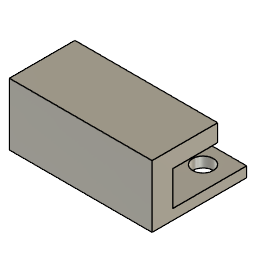
舵机固定 (Autodesk Fusion 360 design; units mm, degrees)
part number: 2025-10-23-15-03-21-135
part number: 2025-10-23-15-21-45-592
Autodesk Fusion 360 part; units mm, degrees
sketch "草图1" plane through (0, 0, 0) normal (0, 0, 1) x (1, 0, 0)
  circle A0 centre (0, 0) radius 1.5
  circle A1 centre (-14, 0) radius 1.5
  line L0 (-14, 0) -> (0, 0) construction
  line L1 (-7, 0) -> (-7, -17.5669) construction
  dimension "d1" = 3
  dimension "d2" = 14
  dimension "d3" = 3
  constraint coincident A0.centre L0.end
  constraint coincident A1.centre L0.start
  constraint horizontal L0
  constraint midpoint L0 L1.start
  constraint perpendicular L0 L1
  measures "d1" diameter of A0
  measures "d2" distance of A1.centre A0.centre
  measures "d3" diameter of A1
sketch "草图2" plane through (0, 0, 0) normal (0, 0, 1) x (1, 0, 0)
  line L0 (-17.3282, -10.7) -> (-17.3282, 3)
  line L1 (-17.3282, 3) -> (3.3282, 3)
  line L2 (3.3282, 3) -> (3.3282, -10.7)
  line L3 (-7, 0) -> (-7, -17.5669)
  line L4 (3.3282, -10.7) -> (-17.3282, -10.7)
  line L5 (-14, 0) -> (0, 0)
  dimension "d4" = 10.7
  dimension "d11" = 3
  constraint vertical L0
  constraint perpendicular L0 L1
  constraint perpendicular L1 L2
  constraint symmetric L0 L2 L3
  constraint perpendicular L0 L4
  measures "d4" distance of L4 L5
  measures "d11" distance of L5.end L1
extrude "拉伸1" add sketch "草图2" along normal blind 1.5 in component "Component'"
extrude "拉伸2" cut sketch "草图1" along normal blind 4 in component "Component'"
sketch "草图4" plane through (0, 0, 1.5) normal (0, 0, 1) x (-1, 0, 0)
  circle A0 centre (14, 0) radius 1.5
  circle A1 centre (0, 0) radius 1.5
  line L0 (-3.3282, 10.7) -> (-3.3282, -3)
  line L1 (-3.3282, -3) -> (17.3282, -3)
  line L2 (17.3282, -3) -> (17.3282, 10.7)
  line L3 (17.3282, 10.7) -> (-3.3282, 10.7)
  line L4 (-3.3282, 10.7) -> (-3.3282, 7.7)
  line L5 (-3.3282, 7.7) -> (17.3282, 7.7)
  line L6 (17.3282, 10.7) -> (-3.3282, 10.7)
  dimension "d12" = 3
  constraint coincident L0.start L3.end
  constraint coincident L0 L4.end
  constraint coincident L2 L5.end
  constraint perpendicular L2 L5
  constraint coincident L2.end L3.start
  measures "d12" distance of L0.start L4.end
extrude "拉伸3" add sketch "草图4" along normal blind 7.5 contours L0 L2 L3 L4 L5 L6 in component "Component'"
sketch "草图5" plane through (0, -7.7, 0) normal (0, 1, 0) x (-1, 0, 0)
  line L0 (-3.3282, 1.5) -> (17.3282, 1.5)
  line L1 (17.3282, 1.5) -> (17.3282, 9)
  line L2 (17.3282, 9) -> (-3.3282, 9)
  line L3 (-3.3282, 9) -> (-3.3282, 1.5)
  line L4 (-3.3282, 6.5) -> (17.3282, 6.5)
  line L5 (17.3282, 9) -> (-3.3282, 9)
  dimension "d15" = 2.5
  constraint coincident L3 L4.start
  constraint coincident L1 L4.end
  constraint perpendicular L1 L4
  constraint coincident L1.end L2.start
  constraint coincident L2.end L3.start
  measures "d15" distance of L4 L5
extrude "拉伸4" add sketch "草图5" along normal blind 6.5 contours L1 L2 L3 L4 L5 in component "Component'"
sketch "草图6" plane through (-17.3282, 0, 0) normal (-1, 0, 0) x (0, -1, 0)
  line L0 (-3, 0) -> (10.7, 0)
  line L1 (10.7, 0) -> (10.7, 9)
  line L2 (10.7, 9) -> (1.2, 9)
  line L3 (1.2, 9) -> (1.2, 6.5)
  line L4 (1.2, 6.5) -> (7.7, 6.5)
  line L5 (7.7, 6.5) -> (7.7, 1.5)
  line L6 (7.7, 1.5) -> (-3, 1.5)
  line L7 (-3, 1.5) -> (-3, 0)
  circle A0 centre (4.7, 7.6) radius 1.05
  point P0 (4.7, 7.6)
  dimension "d18" = 3
  dimension "d19" = 6.1
  dimension "d20" = 2.1
  constraint coincident P0 A0.centre
  measures "d18" distance of L5 P0
  measures "d19" distance of L6 P0
  measures "d20" diameter of A0
extrude "拉伸5" cut sketch "草图6" against normal blind 8.2 contours A0 in component "Component'"
component "Component'" placed x (1, 0, 0) y (0, 1, 0) z (0, 0, 1) at (0, 0, 0)
